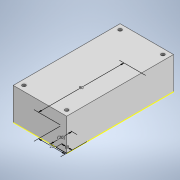
# Autodesk Inventor part: LPS_board
Saved by Autodesk Inventor 2022 (Build 260153000, 153)
## iProperties
Created: 2024-07-06
Part Number: LPS_board
Material: Типовые
Document SubType Name: Modeling
Designer: Капустяник Андрей
Density: 1 g/cm^3
Appearance: По умолчанию
Author: Капустяник Андрей
Autodesk Inventor part; units mm, degrees
ref_plane "YZ Plane" through (0, 0, 0) normal (1, 0, 0) x (0, 1, 0)
ref_plane "XZ Plane" through (0, 0, 0) normal (0, 1, 0) x (-1, 0, 0)
ref_plane "XY Plane" through (0, 0, 0) normal (0, 0, 1) x (1, 0, 0)
sketch "Эскиз1" plane through (0, 0, 0) normal (0, 1, 0) x (-1, 0, 0)
  line L0 (-25, 50) -> (25, 50)
  line L1 (25, 50) -> (25, -50)
  line L2 (25, -50) -> (-25, -50)
  line L3 (-25, -50) -> (-25, 50)
  line L4 (-25, 50) -> (25, -50) construction
  line L5 (25, 50) -> (-25, -50) construction
  point P0 (0, 0)
  dimension "d0" = 50
  dimension "d1" = 100
  constraints: 12 end point, 2 midpoint, 2 parallel, 1 horizontal, 1 perpendicular
  measures "d0" distance of L1.end L2.end
  measures "d1" distance of L0.end L1.end
extrude "Выдавливание1" add sketch "Эскиз1" along normal blind 30
sketch "Эскиз2" plane through (0, 30, 0) normal (0, 1, 0) x (1, 0, 0)
  line L0 (25, 50) -> (-25, 50) projected
  line L1 (-25, 50) -> (-25, -50) projected
  line L2 (-25, -50) -> (25, -50) projected
  line L3 (25, -50) -> (25, 50) projected
  circle A0 centre (20, 45) radius 1.6
  circle A1 centre (20, -45) radius 1.6
  circle A2 centre (-20, -45) radius 1.6
  arc A3 (-20, 52.5) -> (-25, 47.5) centre (-20, 45) ccw projected
  circle A4 centre (-20, 45) radius 1.6
  circle A5 centre (-20, 45) radius 5
  circle A6 centre (20, 45) radius 5
  circle A7 centre (20, -45) radius 5
  circle A8 centre (-20, -45) radius 5
  line L4 (-25, 50) -> (-25, -50) projected
  line L5 (-25, -50) -> (25, -50) projected
  line L6 (25, -50) -> (25, 50) projected
  line L7 (25, 50) -> (-25, 50) projected
  point P0 (0, 0)
  dimension "d5" = 3.2
  dimension "d6" = 3.2
  dimension "d7" = 3.2
  dimension "d8" = 3.2
  dimension "d11" = 10
  dimension "d12" = 10
  dimension "d13" = 10
  dimension "d14" = 10
  constraints: 8 centre point, 8 tangent, 5 coincident, 1 other
  measures "d5" diameter of A0
  measures "d6" diameter of A1
  measures "d7" diameter of A2
  measures "d8" diameter of A4
  measures "d11" diameter of A5
  measures "d12" diameter of A6
  measures "d13" diameter of A7
  measures "d14" diameter of A8
extrude "Выдавливание2" cut sketch "Эскиз2" against normal blind 30 contours A0 | A1 | A2 | A4
sketch "Эскиз3" plane through (0, 0, 0) normal (0, -1, 0) x (1, 0, 0)
  line L0 (25, -50) -> (-25, -50) projected
  line L1 (0, -50) -> (0, 30)
  line L2 (0, 30) -> (25, 30)
  line L3 (25, 50) -> (25, -50) projected
  line L4 (-25, 50) -> (25, 50) projected
  line L5 (25, 50) -> (15, 50)
  line L6 (15, 50) -> (15, 30)
  circle A0 centre (-20, -45) radius 1.6 projected
  circle A1 centre (20, 45) radius 1.6 projected
  circle A2 centre (20, -45) radius 1.6 projected
  circle A3 centre (-20, 45) radius 1.6 projected
  line L7 (25, -50) -> (-25, -50) projected
  line L8 (25, 50) -> (25, -50) projected
  line L9 (-25, 50) -> (25, 50) projected
  line L10 (-25, -50) -> (-25, 50) projected
  point P0 (0, 0)
  dimension "d15" = 80
  dimension "d16" = 25
  dimension "d17" = 10
  dimension "d18" = 20
  constraints: 8 end point, 3 point on line, 1 midpoint, 1 vertical
  measures "d15" distance of L1.start L1.end
  measures "d16" distance of L1.end L2.end
  measures "d17" distance of L3.start L5.end
  measures "d18" distance of L5.end L6.end
sketch "Эскиз4" plane through (-25, 0, -50) normal (-1, 0, 0) x (0, 0, 1)
  point P0 (50, 0)
